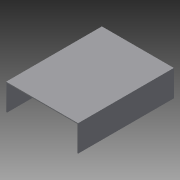
# Autodesk Inventor part: window2
Saved by Autodesk Inventor 2014 SP2 (Build 180246200, 246)
## iProperties
Created: 2016-06-22
Part Number: window2
Material: Generic
Document SubType Name: Modeling
Designer: cruiser
Density: 1 g/cm^3
Appearance: Default
Author: cruiser
Autodesk Inventor part; units mm, degrees
ref_plane "YZ Plane" through (0, 0, 0) normal (1, 0, 0) x (0, 1, 0)
ref_plane "XZ Plane" through (0, 0, 0) normal (0, 1, 0) x (-1, 0, 0)
ref_plane "XY Plane" through (0, 0, 0) normal (0, 0, 1) x (1, 0, 0)
sketch "Sketch1" plane through (0, 0, 0) normal (0, 0, 1) x (1, 0, 0)
  line L0 (-125.5, -166.9563) -> (125.5, -166.9563)
  line L1 (125.5, -166.9563) -> (125.5, 166.9563)
  line L2 (125.5, 166.9563) -> (-125.5, 166.9563)
  line L3 (-125.5, 166.9563) -> (-125.5, -166.9563)
  line L4 (-125.5, -166.9563) -> (125.5, 166.9563) construction
  line L5 (125.5, -166.9563) -> (-125.5, 166.9563) construction
  point P0 (0, 0)
  dimension "d0" = 251
  dimension "d1" = 333.9125
  constraints: 12 end point, 2 midpoint, 2 parallel, 1 horizontal, 1 perpendicular
  measures "d0" distance of L1.end L2.end
  measures "d1" distance of L2.end L0.start
extrude "Extrusion1" add sketch "Sketch1" along normal blind 3.15
sketch "Sketch2" plane through (0, 0, 0) normal (0, 0, -1) x (-1, 0, 0)
  line L0 (125.5, -166.9563) -> (-125.5, -166.9563) projected
  line L1 (-125.5, 166.9563) -> (-122.35, 166.9563)
  line L2 (-122.35, 166.9563) -> (-122.35, -166.9563)
  line L3 (-122.35, -166.9563) -> (-125.5, -166.9563)
  line L4 (-125.5, -166.9563) -> (-125.5, 166.9563)
  line L5 (125.5, 166.9563) -> (122.35, 166.9563)
  line L6 (122.35, 166.9563) -> (122.35, -166.9563)
  line L7 (122.35, -166.9563) -> (125.5, -166.9563)
  line L8 (125.5, -166.9563) -> (125.5, 166.9563)
  line L9 (-122.35, 166.9563) -> (122.35, 166.9563)
  line L10 (122.35, 166.9563) -> (122.35, 163.8062)
  line L11 (122.35, 163.8062) -> (-122.35, 163.8062)
  line L12 (-122.35, 163.8062) -> (-122.35, 166.9563)
  point P0 (0, 0)
  dimension "d4" = 3.15
  dimension "d5" = 3.15
  dimension "d6" = 3.15
  constraints: 24 end point, 6 parallel, 3 horizontal, 3 perpendicular, 3 point on line
  measures "d4" distance of L2.end L3.end
  measures "d5" distance of L7.end L6.end
  measures "d6" distance of L9.end L10.end
extrude "Extrusion2" add sketch "Sketch2" along normal blind 88.65 contours L0 L6 L5 L8 | L0 L4 L1 L2 | L11 L2 L9 L6
equation "\"d0\" = door_x"
equation "\"d1\" = door_z"
equation "\"d2\" = clear_acrylic"
equation "\"d4\" = clear_acrylic"
equation "\"d5\" = clear_acrylic"
equation "\"d6\" = clear_acrylic"
equation "\"d7\" = window_y"
equation "\"sm_thickness\" = 1.5875"
equation "\"al_thickness\" = 1.5875"
equation "\"bend_factor\" = 2.26205"
equation "\"al_bend\" = 3.591"
equation "\"sm_bend\" = 3.591"
equation "\"very_thick_acrylic\" = 9.45"
equation "\"thick_acrylic\" = 5.88"
equation "\"thin_acrylic\" = 3.15"
equation "\"clear_acrylic\" = 3.15"
equation "\"wood_thickness\" = 6.72"
equation "\"m3_diameter\" = 3"
equation "\"m3_head\" = 6"
equation "\"m4_diameter\" = 4"
equation "\"m5_diameter\" = 5"
equation "\"m5_head\" = 10.3"
equation "\"rivet_diameter\" = 3.3"
equation "\"brass_insert_drill\" = 4"
equation "\"m5_brass_insert_drill\" = 6.7"
equation "\"m3_press_nut_drill\" = 4.5"
equation "\"m5_press_nut_drill\" = 6.5"
equation "\"laser_body_diameter\" = 12"
equation "\"carrier_y\" = 251"
equation "\"carrier_y2\" = 76.825"
equation "\"carrier_z\" = 12"
equation "\"carrier_z2\" = 25"
equation "\"visor_x\" = 257.3"
equation "\"visor_y\" = 108.65"
equation "\"window_z\" = 333.9125"
equation "\"window_y\" = 88.65"
equation "\"window_overlap\" = 48"
equation "\"acrylic_into_frame\" = 5"
equation "\"door_x\" = 251"
equation "\"door_z\" = 333.9125"
equation "\"door_overlap\" = 48"
equation "\"reservoir_x\" = 201"
equation "\"reservoir_y\" = 201"
equation "\"linear_bearing_spacing\" = 271"
equation "\"tray_border\" = 25"
equation "\"tray_x\" = 251"
equation "\"tray_y\" = 251"
equation "\"bed_z\" = 25"
equation "\"crane_z2\" = 12"
equation "\"switch_spacing\" = 19"
equation "\"frame_top_z\" = 385"
equation "\"frame_bottom_z\" = 275"
equation "\"frame_total_z\" = 661.5875"
equation "\"frame_x\" = 350.2"
equation "\"frame_face_y\" = 45"
equation "\"frame_border\" = 46.35"
equation "\"frame_foot_z\" = 12"
equation "\"frame_screw_from_center\" = 25"
equation "\"laser_y_offset\" = 19.4"
equation "\"laser_diameter\" = 12"
equation "\"laser_z_offset\" = 55"
equation "\"laser_y\" = 15"
equation "\"laser_z\" = 75"
equation "\"laser_gap\" = 1"
equation "\"subframe_x\" = 66"
equation "\"subframe_y\" = 55"
equation "\"galvo_frame_x\" = 66"
equation "\"galvo_frame_z\" = 65"
equation "\"galvo_frame_y_offset\" = 27.5"
equation "\"drawer_x\" = 257.3"
equation "\"drawer_y\" = 85.2375"
equation "\"drawer_z\" = 278.175"
equation "\"drawer_support_from_top\" = 48"
equation "\"drawer_screw_z\" = 145"
equation "\"drawer_screw_from_center\" = 55"
equation "\"nema17_x\" = 43"
body "Solid1"
